# Autodesk Inventor part: BS 4320 - M30 (Form E)
Saved by Autodesk Inventor 2020.1 (Build 241239000, 239)
## iProperties
Comments: To add or edit properties for Autodesk Inventor files, use iProperties.
Shininess: 64.0
Length Units: 11269
Angle Units: 11279
Time Units: 11290
Mass Units: 11283
Length Display Precision: 3
Angle Display Precision: 2
Compacted: True
Alert: To add or edit properties for Autodesk Inventor files, use iProperties.
Created: 2003-05-03
Part Number: BS 4320 - M30 (Form E)
Vendor: Autodesk Inc.
Document SubType Name: Modeling
Designer: Stephen Hooper
Material: Generic
Description: Black Washer
Standard: BS 4320
Manufacturer: Standard
Standards Organization: Custom
Density: 1 g/cm^3
Appearance: Default
Density: 0.0
Volumn: 0.0
Area: 0.0
PropertySet Name: Model Information
Control State: 0
Master: False
Checked Out: False
Author: Stephen Hooper
Revision Number: 5
Autodesk Inventor part; units mm, degrees
ref_plane "YZ Plane" through (0, 0, 0) normal (1, 0, 0) x (0, 1, 0)
ref_plane "XZ Plane" through (0, 0, 0) normal (0, 1, 0) x (-1, 0, 0)
ref_plane "XY Plane" through (0, 0, 0) normal (0, 0, 1) x (1, 0, 0)
sketch "Sketch" plane through (0, 0, 0) normal (1, 0, 0) x (0, 1, 0)
  circle A0 centre (0, 0) radius 28
  circle A1 centre (0, 0) radius 16.5
  dimension "d0" = 33
  dimension "d1" = 56
  constraints: 2 centre point, 2 coincident
  measures "d0" diameter of A1
  measures "d1" diameter of A0
extrude "Body" add sketch "Sketch" along normal blind 4
equation "\"d0\" = SD1"
equation "\"d1\" = SD2"
equation "\"d2\" = SD"
equation "\"SD1\" = 33"
equation "\"SD2\" = 56"
equation "\"SD\" = 4"
body "Solid1"
